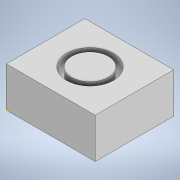
# Autodesk Inventor part: CameraOverhead
Saved by Autodesk Inventor 2020.3 (Build 243373000, 373)
## iProperties
Created: 2020-06-08
Part Number: CameraOverhead
Material: Generic
Document SubType Name: Modeling
Designer: super
Density: 1 g/cm^3
Appearance: Default
Author: super
Autodesk Inventor part; units mm, degrees
ref_plane "YZ Plane" through (0, 0, 0) normal (1, 0, 0) x (0, 1, 0)
ref_plane "XZ Plane" through (0, 0, 0) normal (0, 1, 0) x (-1, 0, 0)
ref_plane "XY Plane" through (0, 0, 0) normal (0, 0, 1) x (1, 0, 0)
sketch "Sketch1" plane through (0, 0, 0) normal (0, 1, 0) x (-1, 0, 0)
  point P0 (0, 0)
sketch "Sketch2" plane through (0, 0, 0) normal (0, 1, 0) x (-1, 0, 0)
  line L0 (0, 0) -> (-51, 0)
  line L1 (-51, 0) -> (-51, -45)
  line L2 (-51, -45) -> (0, -45)
  line L3 (0, 0) -> (0, -45)
  line L4 (0, -45) -> (0, -22.5)
  circle A0 centre (-21.5, -22.5) radius 12.5
  dimension "d0" = 51
  dimension "d1" = 45
  dimension "d6" = 25
  constraints: 10 end point, 1 centre point, 1 horizontal, 1 midpoint, 1 parallel, 1 perpendicular, 1 vertical
  measures "d0" distance of L2.end L1.end
  measures "d1" distance of L1.end L0.end
  measures "d6" diameter of A0
extrude "Extrusion1" add sketch "Sketch2" along normal blind 11
sketch "Sketch3" plane through (0, 11, 0) normal (0, 1, 0) x (1, 0, 0)
  line L0 (0, 45) -> (0, 0) projected
  line L1 (51, 0) -> (51, 45) projected
  line L2 (0, 0) -> (51, 0)
  line L3 (51, 0) -> (51, 45)
  line L4 (51, 45) -> (0, 45)
  line L5 (0, 45) -> (0, 0)
  constraints: 8 end point, 2 parallel, 1 horizontal, 1 perpendicular
extrude "Extrusion2" add sketch "Sketch3" along normal blind 12
sketch "Sketch4" plane through (0, 23, 0) normal (0, 1, 0) x (1, 0, 0)
  line L0 (0, 45) -> (0, 0) projected
  line L1 (0, 0) -> (51, 0) projected
  line L2 (3, 14) -> (3, 31)
  line L3 (3, 22.5) -> (3, 20.3)
  line L4 (3, 20.3) -> (3, 24.7)
  line L5 (17.5, 19.5) -> (3, 20.3)
  line L6 (3, 24.7) -> (17.5, 25.5)
  line L7 (17.5, 25.5) -> (17.5, 31.5)
  line L8 (17.5, 31.5) -> (21.5, 31.5)
  line L9 (21.5, 31.5) -> (21.5, 26.5)
  line L10 (17.5, 19.5) -> (17.5, 13.5)
  line L11 (17.5, 13.5) -> (21.5, 13.5)
  line L12 (21.5, 13.5) -> (21.5, 18.5)
  line L13 (38.5, 22.5) -> (38.5, 20.3)
  line L14 (38.5, 20.3) -> (38.5, 24.7)
  line L15 (38.5, 24.7) -> (21.5, 26.5)
  line L16 (38.5, 20.3) -> (21.5, 18.5)
  dimension "d13" = 17
  dimension "d14" = 2.2
  dimension "d15" = 4.4
  dimension "d18" = 6
  dimension "d19" = 6
  dimension "d20" = 4
  dimension "d21" = 5
  dimension "d23" = 6
  dimension "d24" = 4
  dimension "d25" = 5
  dimension "d26" = 2.2
  dimension "d27" = 4.4
  constraints: 30 end point, 4 perpendicular, 3 point on line, 3 vertical, 1 midpoint
  measures "d13" distance of L2.start L2.end
  measures "d14" distance of L3.start L3.end
  measures "d15" distance of L3.end L4.end
  measures "d18" distance of L6.end L5.start
  measures "d19" distance of L6.end L7.end
  measures "d20" distance of L7.end L8.end
  measures "d21" distance of L8.end L9.end
  measures "d23" distance of L5.start L10.end
  measures "d24" distance of L10.end L11.end
  measures "d25" distance of L11.end L12.end
  measures "d26" distance of L13.start L13.end
  measures "d27" distance of L13.end L14.end
extrude "Extrusion3" cut sketch "Sketch4" against normal blind 4
extrude "Extrusion4" add sketch "Sketch4" against normal blind 4
sketch "Sketch5" plane through (0, 23, 0) normal (0, 1, 0) x (1, 0, 0)
  line L0 (0, 0) -> (51, 0) projected
  circle A0 centre (25.5, 22.5) radius 13.5
  circle A1 centre (25.5, 22.5) radius 10.5
  dimension "d32" = 27
  dimension "d33" = 21
  constraints: 2 centre point, 1 coincident
  measures "d32" diameter of A0
  measures "d33" diameter of A1
extrude "Extrusion5" cut sketch "Sketch5" against normal blind 15
sketch "Sketch6" plane through (0, 0, 0) normal (0, -1, 0) x (1, 0, 0)
  arc A0 (20.25, -34.9373) -> (29.25, -32.3075) centre (21.5, -22.5) ccw projected
  circle A1 centre (21.5, -22.5) radius 12.5
  point P0 (0, 0)
  constraints: 1 centre point, 1 coincident
extrude "Extrusion6" add sketch "Sketch6" against normal blind 11
sketch "Sketch7" plane through (0, 0, 0) normal (0, -1, 0) x (1, 0, 0)
  line L0 (21.5, -27) -> (34, -27)
  line L1 (34, -27) -> (34, -22.5)
  line L2 (34, -22.5) -> (34, -18)
  line L3 (34, -18) -> (9, -18)
  line L4 (9, -18) -> (9, -27)
  line L5 (9, -27) -> (21.5, -27)
  circle A0 centre (21.5, -22.5) radius 12.5
  point P0 (0, 0)
  point P1 (33.1619, -18)
  point P2 (9.8381, -18)
  point P3 (9.8381, -27)
  point P4 (33.1619, -27)
  dimension "d44" = 12.5
  dimension "d45" = 4.5
  dimension "d46" = 25
  dimension "d47" = 9
  dimension "d48" = 25
  constraints: 12 end point, 3 perpendicular, 2 point on line, 1 centre point
  measures "d44" distance of L0.start L0.end
  measures "d45" distance of L1.end L2.end
  measures "d46" distance of L2.end L3.end
  measures "d47" distance of L3.end L4.end
  measures "d48" diameter of A0
extrude "Extrusion7" cut sketch "Sketch7" against normal blind 11 contours L5 A0 L3 L0
body "Solid1"
